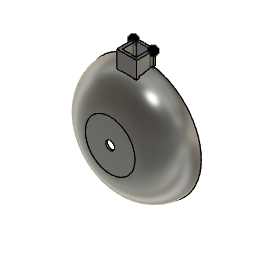
dumb_doorbell v1 (Autodesk Fusion 360 design; units mm, degrees)
Autodesk Fusion 360 part; units mm, degrees
sketch "Sketch1" plane through (0, 0, 0) normal (0, 0, 1) x (1, 0, 0)
  line L0 (0, 0) -> (15.001, 0)
  line L1 (35, 19.999) -> (35, 20)
  arc A0 (15.001, 0) -> (35, 19.999) centre (15.001, 19.999) ccw
  line L2 (0, 1) -> (15.001, 1)
  arc A1 (15.001, 1) -> (34, 19.999) centre (15.001, 19.999) ccw
  line L3 (34, 19.999) -> (34, 20)
  line L4 (34, 20) -> (35, 20)
  line L5 (0, 1) -> (0, 0)
  point P0 (35, 0)
  dimension "d1" = 35
  dimension "d2" = 20
  dimension "d3" = 19.999
  dimension "d4" = -1
  constraint horizontal L0
  constraint vertical L1
  constraint coincident L0.start L5.end
  constraint coincident P0 L1
  constraint coincident P0 L0
  constraint tangent L1 A0
  constraint tangent L0 A0
  constraint perpendicular L1 L4
  constraint perpendicular L0 L5
  measures "d1" distance of L0.start P0
  measures "d2" distance of P0 L1.end
  measures "d3" radius of A0
revolve "Revolve1" add sketch "Sketch1" angle 360 about axis through (0, 1.75, 0) along (0, 1, 0)
ref_plane "WorkPlane1" through (0, 0, 35) normal (0, 0, 1) x (1, 0, 0)
sketch "Sketch2" plane through (0, 0, 35) normal (0, 0, 1) x (1, 0, 0)
  line L0 (0, 0) -> (0, 15.5)
  circle A0 centre (0, 15.5) radius 2.05
  dimension "d7" = 15.5
  dimension "d8" = 4.1
  constraint coincident L0.start origin
  constraint vertical L0
  constraint coincident L0.end A0.centre
  measures "d7" distance of L0.start L0.end
  measures "d8" diameter of A0
extrude "Extrude1" cut sketch "Sketch2" against normal blind 10
sketch "Sketch3" plane through (0, 0, 0) normal (0, -1, 0) x (1, 0, 0)
  circle A0 centre (0, 0) radius 15.001
  circle A1 centre (0, 0) radius 2.65
  dimension "d11" = 5.3
  constraint coincident A0.centre A1.centre
  measures "d11" diameter of A1
extrude "Extrude2" cut sketch "Sketch3" along normal blind 30 and the other way blind 30 contours A1
sketch "Sketch4" plane through (0, 20, 0) normal (0, 1, 0) x (-1, 0, 0)
  circle A0 centre (0, 0) radius 34
  circle A1 centre (0, 0) radius 35
  line L0 (-6, 42.4664) -> (6, 42.4664)
  line L1 (6, 42.4664) -> (6, 33.4664)
  line L2 (-6, 33.4664) -> (-6, 42.4664)
  line L3 (-6, 42.4664) -> (0, 34) construction
  line L4 (6, 42.4664) -> (0, 34) construction
  line L5 (0, 34) -> (-6, 34)
  line L6 (0, 34) -> (6, 34)
  dimension "d16" = 9
  dimension "d19" = 12
  dimension "d20" = 6
  constraint horizontal L0
  constraint perpendicular L0 L1
  constraint parallel L1 L2
  constraint coincident A0 L3.end
  constraint coincident L3.end L4.end
  constraint coincident A0 L1.end
  constraint coincident L1 L6.end
  constraint coincident A0 L2.start
  constraint coincident L2 L5.end
  measures "d16" distance of L0.start L2.start
  measures "d19" distance of L0.start L0.end
  measures "d20" distance of L2 L3.end
extrude "Extrude3" add sketch "Sketch4" along normal blind 1.5 contours A1 L1 L2 L5 L6 | A1 L0 L1 L2
sketch "Sketch5" plane through (0, 20, 0) normal (0, -1, 0) x (1, 0, 0)
  arc A0 (6, 34.4819) -> (-6, 34.4819) centre (0, 0) ccw
  line L0 (6, 34.4819) -> (6, 42.4664)
  line L1 (6, 42.4664) -> (-6, 42.4664)
  line L2 (-6, 42.4664) -> (-6, 34.4819)
  line L3 (6, 42.4664) -> (4.25, 42.4664)
  line L4 (4.25, 42.4664) -> (4.25, 33.4664)
  line L5 (4.25, 33.4664) -> (6, 33.4664)
  line L6 (6, 33.4664) -> (6, 42.4664)
  line L7 (-6, 42.4664) -> (-4.25, 42.4664)
  line L8 (-4.25, 42.4664) -> (-4.25, 33.4664)
  line L9 (-4.25, 33.4664) -> (-6, 33.4664)
  line L10 (-6, 33.4664) -> (-6, 42.4664)
  dimension "d21" = 9
  dimension "d22" = 1.75
  dimension "d23" = 1.75
  dimension "d24" = 9
  constraint horizontal L3
  constraint vertical L4
  constraint horizontal L5
  constraint vertical L6
  constraint coincident L0.end L1.start
  constraint horizontal L7
  constraint vertical L8
  constraint horizontal L9
  constraint vertical L10
  constraint coincident L1.end L2.start
  measures "d21" distance of L0.end L5.end
  measures "d22" distance of L0.end L3.end
  measures "d23" distance of L1.end L7.end
  measures "d24" distance of L1.end L9.end
extrude "Extrude4" add sketch "Sketch5" along normal blind 8 contours A0 L0 L1 L3 L4 L6 | A0 L1 L2 L7 L8 L10
extrude "Extrude5" cut sketch "Sketch5" along normal blind 8 contours A0 L4 L5 L6 | A0 L0 L1 L3 L4 L6 | A0 L8 L9 L10 | A0 L1 L2 L7 L8 L10
extrude "Extrude6" add sketch "Sketch5" along normal blind 8 contours A0 L4 L5 L6 | A0 L0 L1 L3 L4 L6 | A0 L8 L9 L10 | A0 L1 L2 L7 L8 L10
extrude "Extrude7" add sketch "Sketch5" along normal blind 8.5 contours A0 L4 L5 L6 | A0 L0 L1 L3 L4 L6 | A0 L8 L9 L10 | A0 L1 L2 L7 L8 L10
sketch "Sketch6" plane through (0, 11.5, 0) normal (0, -1, 0) x (1, 0, 0)
  line L0 (6, 33.4664) -> (6, 42.4664)
  line L1 (6, 42.4664) -> (4.25, 42.4664)
  line L2 (4.25, 42.4664) -> (4.25, 33.4664)
  line L3 (4.25, 33.4664) -> (6, 33.4664)
  line L4 (6, 42.4664) -> (-6, 42.4664)
  line L5 (-6, 42.4664) -> (-6, 32)
  line L6 (-6, 32) -> (6, 32)
  line L7 (6, 32) -> (6, 42.4664)
  constraint horizontal L4
  constraint vertical L5
  constraint horizontal L6
  constraint vertical L7
  constraint coincident L0.end L1.start
extrude "Extrude8" add sketch "Sketch6" along normal blind 1.5
